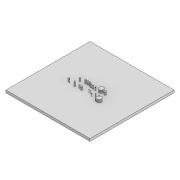
# Autodesk Inventor part: scene7
Saved by Autodesk Inventor 2021 (Build 250183000, 183)
## iProperties
Created: 2022-04-06
Part Number: scene7
Material: Generic
Document SubType Name: Modeling
Designer: Derm
Density: 1 g/cm^3
Appearance: Default
Author: Derm
Autodesk Inventor part; units mm, degrees
ref_plane "YZ Plane" through (0, 0, 0) normal (1, 0, 0) x (0, 1, 0)
ref_plane "XZ Plane" through (0, 0, 0) normal (0, 1, 0) x (-1, 0, 0)
ref_plane "XY Plane" through (0, 0, 0) normal (0, 0, 1) x (1, 0, 0)
sketch "Sketch1" plane through (0, 0, 0) normal (0, 1, 0) x (-1, 0, 0)
  line L0 (-50000, 50000) -> (50000, 50000)
  line L1 (50000, 50000) -> (50000, -50000)
  line L2 (50000, -50000) -> (-50000, -50000)
  line L3 (-50000, -50000) -> (-50000, 50000)
  line L4 (-50000, 50000) -> (50000, -50000) construction
  line L5 (50000, 50000) -> (-50000, -50000) construction
  point P0 (0, 0)
  dimension "d0" = 100000
  dimension "d1" = 100000
  constraints: 12 end point, 2 midpoint, 2 parallel, 1 horizontal, 1 perpendicular
  measures "d0" distance of L1.end L2.end
  measures "d1" distance of L0.end L1.end
extrude "Extrusion1" add sketch "Sketch1" against normal blind 3000
sketch "Sketch2" plane through (0, 0, 0) normal (0, 1, 0) x (1, 0, 0)
  line L0 (50000, 50000) -> (-50000, 50000) projected
  line L1 (-50000, 50000) -> (-50000, -50000) projected
  line L2 (-50000, -50000) -> (50000, -50000) projected
  line L3 (50000, -50000) -> (50000, 50000) projected
  line L4 (50000, 50000) -> (50000, -50000) projected
  line L5 (-50000, -2000) -> (50000, -2000)
  line L6 (50000, -2000) -> (50000, 2000)
  line L7 (50000, 2000) -> (-50000, 2000)
  line L8 (-50000, 2000) -> (-50000, -2000)
  line L9 (-50000, -2000) -> (50000, 2000) construction
  line L10 (50000, -2000) -> (-50000, 2000) construction
  line L11 (5190.5361, 8455.2241) -> (11345.2122, 8455.2241)
  line L12 (11345.2122, 8455.2241) -> (11345.2122, 2832.4339)
  line L13 (11345.2122, 2832.4339) -> (5190.5361, 2832.4339)
  line L14 (5190.5361, 2832.4339) -> (5190.5361, 8455.2241)
  line L15 (5190.5361, 8455.2241) -> (11345.2122, 2832.4339) construction
  line L16 (11345.2122, 8455.2241) -> (5190.5361, 2832.4339) construction
  line L17 (13548.7384, -7995.2366) -> (20995.1366, -7995.2366)
  line L18 (20995.1366, -7995.2366) -> (20995.1366, -2828.3483)
  line L19 (20995.1366, -2828.3483) -> (13548.7384, -2828.3483)
  line L20 (13548.7384, -2828.3483) -> (13548.7384, -7995.2366)
  line L21 (13548.7384, -7995.2366) -> (20995.1366, -2828.3483) construction
  line L22 (20995.1366, -7995.2366) -> (13548.7384, -2828.3483) construction
  line L23 (593.5251, -2562.4055) -> (4772.6262, -2562.4055)
  line L24 (4772.6262, -2562.4055) -> (4772.6262, -3778.1439)
  line L25 (4772.6262, -3778.1439) -> (593.5251, -3778.1439)
  line L26 (593.5251, -3778.1439) -> (593.5251, -2562.4055)
  line L27 (593.5251, -2562.4055) -> (4772.6262, -3778.1439) construction
  line L28 (4772.6262, -2562.4055) -> (593.5251, -3778.1439) construction
  line L29 (-10538.0803, 5605.837) -> (-4079.4695, 5605.837)
  line L30 (-4079.4695, 5605.837) -> (-4079.4695, 3706.2457)
  line L31 (-4079.4695, 3706.2457) -> (-10538.0803, 3706.2457)
  line L32 (-10538.0803, 3706.2457) -> (-10538.0803, 5605.837)
  line L33 (-10538.0803, 5605.837) -> (-4079.4695, 3706.2457) construction
  line L34 (-4079.4695, 5605.837) -> (-10538.0803, 3706.2457) construction
  line L35 (-3357.6248, 4314.115) -> (1581.3128, 4314.115)
  line L36 (1581.3128, 4314.115) -> (1581.3128, 2642.4746)
  line L37 (1581.3128, 2642.4746) -> (-3357.6248, 2642.4746)
  line L38 (-3357.6248, 2642.4746) -> (-3357.6248, 4314.115)
  line L39 (-3357.6248, 4314.115) -> (1581.3128, 2642.4746) construction
  line L40 (1581.3128, 4314.115) -> (-3357.6248, 2642.4746) construction
  line L41 (-9040.7205, -3304.0821) -> (-4779.0471, -3304.0821)
  line L42 (-4779.0471, -3304.0821) -> (-4779.0471, -6275.5798)
  line L43 (-4779.0471, -6275.5798) -> (-9040.7205, -6275.5798)
  line L44 (-9040.7205, -6275.5798) -> (-9040.7205, -3304.0821)
  line L45 (-9040.7205, -3304.0821) -> (-4779.0471, -6275.5798) construction
  line L46 (-4779.0471, -3304.0821) -> (-9040.7205, -6275.5798) construction
  line L47 (12978.8612, 2832.4339) -> (15790.2565, 4086.164)
  line L48 (15790.2565, 4086.164) -> (14919.446, 6038.8907)
  line L49 (14919.446, 6038.8907) -> (12108.0508, 4785.1606)
  line L50 (12108.0508, 4785.1606) -> (12978.8612, 2832.4339)
  line L51 (7237.4094, -5991.9062) -> (11076.909, -4432.894)
  line L52 (11076.909, -4432.894) -> (10571.8855, -3189.1337)
  line L53 (10571.8855, -3189.1337) -> (6732.3859, -4748.1459)
  line L54 (6732.3859, -4748.1459) -> (7237.4094, -5991.9062)
  line L55 (-16072.161, 3808.7972) -> (-15391.3811, 2832.4339)
  line L56 (-15391.3811, 2832.4339) -> (-14124.812, 3715.5628)
  line L57 (-14124.812, 3715.5628) -> (-14805.5919, 4691.9262)
  line L58 (-14805.5919, 4691.9262) -> (-16072.161, 3808.7972)
  line L59 (-23491.5084, -4748.1459) -> (-20999.8327, -7024.4914)
  line L60 (-20999.8327, -7024.4914) -> (-18908.6968, -4735.5451)
  line L61 (-18908.6968, -4735.5451) -> (-21400.3724, -2459.1996)
  line L62 (-21400.3724, -2459.1996) -> (-23491.5084, -4748.1459)
  line L63 (-16105.7388, -3167.2582) -> (-12909.355, -5395.9713)
  line L64 (-12909.355, -5395.9713) -> (-12180.8401, -4351.1472)
  line L65 (-12180.8401, -4351.1472) -> (-15377.224, -2122.4342)
  line L66 (-15377.224, -2122.4342) -> (-16105.7388, -3167.2582)
  line L67 (2445.7903, 4086.164) -> (3479.5334, 2000)
  line L68 (3479.5334, 2000) -> (4246.1072, 2379.8553)
  line L69 (4246.1072, 2379.8553) -> (3212.3641, 4466.0192)
  line L70 (3212.3641, 4466.0192) -> (2445.7903, 4086.164)
  point P0 (0, 0)
  point P1 (8267.8742, 5643.829)
  point P2 (17271.9375, -5411.7924)
  point P3 (2683.0756, -3170.2747)
  point P4 (-7308.7749, 4656.0414)
  point P5 (-888.156, 3478.2948)
  point P6 (-6909.8838, -4789.831)
  dimension "d4" = 4000
  constraints: 132 end point, 27 parallel, 14 midpoint, 13 perpendicular, 7 horizontal, 3 point on line
  measures "d4" distance between parallel lines of L7 L5
extrude "Extrusion2" add sketch "Sketch2" along normal blind 3000 contours L67 L70 L69 L68 | L11 L12 L13 L14 | L20 L19 L18 L17 | L23 L24 L25 L26 | L29 L30 L31 L32 | L35 L36 L37 L38 | L41 L42 L43 L44 | L50 L49 L48 L47 | L54 L53 L52 L51 | L58 L57 L56 L55 | L62 L61 L60 L59 | L66 L65 L64 L63
fillet "Fillet1" [suppressed]
sketch "Sketch3" plane through (0, 0, 0) normal (0, 1, 0) x (1, 0, 0)
  line L0 (-9040.7205, -6275.5798) -> (-9040.7205, -3304.0821) projected
  line L1 (-9040.7205, -3304.0821) -> (-4779.0471, -3304.0821) projected
  line L2 (-4779.0471, -3304.0821) -> (-4779.0471, -6275.5798) projected
  line L3 (-4779.0471, -6275.5798) -> (-9040.7205, -6275.5798) projected
  line L4 (593.5251, -3778.1439) -> (593.5251, -2562.4055) projected
  line L5 (593.5251, -2562.4055) -> (4772.6262, -2562.4055) projected
  line L6 (4772.6262, -2562.4055) -> (4772.6262, -3778.1439) projected
  line L7 (4772.6262, -3778.1439) -> (593.5251, -3778.1439) projected
  line L8 (15790.2565, 4086.164) -> (12978.8612, 2832.4339) projected
  line L9 (12978.8612, 2832.4339) -> (12108.0508, 4785.1606) projected
  line L10 (12108.0508, 4785.1606) -> (14919.446, 6038.8907) projected
  line L11 (14919.446, 6038.8907) -> (15790.2565, 4086.164) projected
  line L12 (5190.5361, 2832.4339) -> (5190.5361, 8455.2241) projected
  line L13 (5190.5361, 8455.2241) -> (11345.2122, 8455.2241) projected
  line L14 (11345.2122, 8455.2241) -> (11345.2122, 2832.4339) projected
  line L15 (11345.2122, 2832.4339) -> (5190.5361, 2832.4339) projected
  line L16 (-3357.6248, 2642.4746) -> (-3357.6248, 4314.115) projected
  line L17 (-3357.6248, 4314.115) -> (1581.3128, 4314.115) projected
  line L18 (1581.3128, 4314.115) -> (1581.3128, 2642.4746) projected
  line L19 (1581.3128, 2642.4746) -> (-3357.6248, 2642.4746) projected
  line L20 (-12909.355, -5395.9713) -> (-16105.7388, -3167.2582) projected
  line L21 (-16105.7388, -3167.2582) -> (-15377.224, -2122.4342) projected
  line L22 (-15377.224, -2122.4342) -> (-12180.8401, -4351.1472) projected
  line L23 (-12180.8401, -4351.1472) -> (-12909.355, -5395.9713) projected
  line L24 (-15391.3811, 2832.4339) -> (-16072.161, 3808.7972) projected
  line L25 (-16072.161, 3808.7972) -> (-14805.5919, 4691.9262) projected
  line L26 (-14805.5919, 4691.9262) -> (-14124.812, 3715.5628) projected
  line L27 (-14124.812, 3715.5628) -> (-15391.3811, 2832.4339) projected
  line L28 (11076.909, -4432.894) -> (7237.4094, -5991.9062) projected
  line L29 (7237.4094, -5991.9062) -> (6732.3859, -4748.1459) projected
  line L30 (6732.3859, -4748.1459) -> (10571.8855, -3189.1337) projected
  line L31 (10571.8855, -3189.1337) -> (11076.909, -4432.894) projected
  line L32 (20995.1366, -7995.2366) -> (13548.7384, -7995.2366) projected
  line L33 (13548.7384, -7995.2366) -> (13548.7384, -2828.3483) projected
  line L34 (13548.7384, -2828.3483) -> (20995.1366, -2828.3483) projected
  line L35 (20995.1366, -2828.3483) -> (20995.1366, -7995.2366) projected
  line L36 (2445.7903, 4086.164) -> (3212.3641, 4466.0192) projected
  line L37 (3212.3641, 4466.0192) -> (4246.1072, 2379.8553) projected
  line L38 (4246.1072, 2379.8553) -> (3479.5334, 2000) projected
  line L39 (3479.5334, 2000) -> (2445.7903, 4086.164) projected
  line L40 (-10538.0803, 3706.2457) -> (-10538.0803, 5605.837) projected
  line L41 (-10538.0803, 5605.837) -> (-4079.4695, 5605.837) projected
  line L42 (-4079.4695, 5605.837) -> (-4079.4695, 3706.2457) projected
  line L43 (-4079.4695, 3706.2457) -> (-10538.0803, 3706.2457) projected
  line L44 (-20999.8327, -7024.4914) -> (-23491.5084, -4748.1459) projected
  line L45 (-23491.5084, -4748.1459) -> (-21400.3724, -2459.1996) projected
  line L46 (-21400.3724, -2459.1996) -> (-18908.6968, -4735.5451) projected
  line L47 (-18908.6968, -4735.5451) -> (-20999.8327, -7024.4914) projected
  line L48 (50000, 50000) -> (-50000, 50000) projected
  line L49 (-50000, 50000) -> (-50000, -50000) projected
  line L50 (-50000, -50000) -> (50000, -50000) projected
  line L51 (50000, -50000) -> (50000, 50000) projected
  circle A0 centre (-21206.9989, -4735.5451) radius 2507.8736
  circle A1 centre (-14179.4153, -3811.0138) radius 1948.3346
  line L52 (-15377.224, -2122.4342) -> (-16105.7388, -3167.2582) projected
  circle A2 centre (-15130.9909, 3808.7972) radius 991.1752
  line L53 (-10538.0803, 3706.2457) -> (-10538.0803, 5605.837) projected
  circle A3 centre (-7308.7749, 7370.1362) radius 4883.9028
  line L54 (1581.3128, 2642.4746) -> (-3357.6248, 2642.4746) projected
  circle A4 centre (-888.156, 6827.5495) radius 4859.3341
  line L55 (4246.1072, 2379.8553) -> (3479.5334, 2000) projected
  circle A5 centre (3345.9488, 3233.0096) radius 1240.2248
  line L56 (5190.5361, 2832.4339) -> (5190.5361, 8455.2241) projected
  circle A6 centre (8267.8742, 8184.0163) radius 6173.2847
  circle A7 centre (14033.4063, 4473.2344) radius 1950.4594
  line L57 (10571.8855, -3189.1337) -> (6732.3859, -4748.1459) projected
  circle A8 centre (8880.1815, -4432.894) radius 2099.7148
  line L58 (4772.6262, -2562.4055) -> (4772.6262, -3778.1439) projected
  circle A9 centre (2683.0756, -3170.2747) radius 2176.1724
  circle A10 centre (-6909.8838, -4789.831) radius 2597.6749
  line L59 (13548.7384, -7995.2366) -> (13548.7384, -2828.3483) projected
  circle A11 centre (16975.0214, -4873.5592) radius 3990.2761
  point P0 (0, 0)
  point P1 (12325.3726, 3531.4739)
  point P2 (14183.1434, 6417.9376)
  point P3 (-16034.8819, -3216.664)
  point P4 (-12980.2119, -5346.5655)
  point P5 (-12287.5612, -4276.7348)
  point P6 (-15270.5029, -2196.8466)
  constraints: 3 centre point, 1 tangent, 27 other
extrude "Extrusion3" [suppressed]
sketch "Sketch4" plane through (0, 0, 0) normal (0, 1, 0) x (1, 0, 0)
  line L0 (50000, 50000) -> (-50000, 50000) projected
  line L1 (-50000, 50000) -> (-50000, -50000) projected
  line L2 (-50000, -50000) -> (50000, -50000) projected
  line L3 (50000, -50000) -> (50000, 50000) projected
  line L4 (11076.909, -4432.894) -> (7237.4094, -5991.9062) projected
  line L5 (7237.4094, -5991.9062) -> (6732.3859, -4748.1459) projected
  line L6 (6732.3859, -4748.1459) -> (10571.8855, -3189.1337) projected
  line L7 (10571.8855, -3189.1337) -> (11076.909, -4432.894) projected
  line L8 (-10538.0803, 3706.2457) -> (-10538.0803, 5605.837) projected
  line L9 (-10538.0803, 5605.837) -> (-4079.4695, 5605.837) projected
  line L10 (-14805.5919, 4691.9262) -> (-14124.812, 3715.5628) projected
  line L11 (-14124.812, 3715.5628) -> (-15391.3811, 2832.4339) projected
  line L12 (-15391.3811, 2832.4339) -> (-16072.161, 3808.7972) projected
  line L13 (593.5251, -3778.1439) -> (593.5251, -2562.4055) projected
  line L14 (4772.6262, -2562.4055) -> (4772.6262, -3778.1439) projected
  line L15 (20995.1366, -7995.2366) -> (13548.7384, -7995.2366) projected
  line L16 (13548.7384, -7995.2366) -> (13548.7384, -2828.3483) projected
  line L17 (13548.7384, -2828.3483) -> (20995.1366, -2828.3483) projected
  line L18 (20995.1366, -2828.3483) -> (20995.1366, -7995.2366) projected
  line L19 (-12909.355, -5395.9713) -> (-16105.7388, -3167.2582) projected
  line L20 (-16105.7388, -3167.2582) -> (-15377.224, -2122.4342) projected
  line L21 (-15377.224, -2122.4342) -> (-12180.8401, -4351.1472) projected
  line L22 (-12180.8401, -4351.1472) -> (-12909.355, -5395.9713) projected
  circle A0 centre (-4095.3087, 1822.3221) radius 119.7331
  circle A1 centre (-3557.0154, -1685.8651) radius 153.3297
  circle A2 centre (1083.4441, 1432.5236) radius 98.3053
  circle A3 centre (5092.8011, 1785.6866) radius 131.4219
  circle A4 centre (5747.1243, -1847.542) radius 169.4608
  circle A5 centre (9343.4621, 1432.5236) radius 127.5966
  circle A6 centre (-7082.9402, 1822.3221) radius 106.718
  circle A7 centre (-7308.7749, -1847.542) radius 87.1079
  circle A8 centre (-10330.2163, 2528.7629) radius 78.0049
  circle A9 centre (-11168.7148, -2334.5281) radius 88.8954
  circle A10 centre (-13446.3785, 2742.5645) radius 100.7642
  line L23 (593.5251, -2562.4055) -> (4772.6262, -2562.4055) projected
  line L24 (4772.6262, -3778.1439) -> (593.5251, -3778.1439) projected
  line L25 (-16072.161, 3808.7972) -> (-14805.5919, 4691.9262) projected
  line L26 (-4079.4695, 5605.837) -> (-4079.4695, 3706.2457) projected
  line L27 (-4079.4695, 3706.2457) -> (-10538.0803, 3706.2457) projected
  point P0 (0, 0)
  constraints: 11 centre point
extrude "Extrusion4" [suppressed]
sketch "Sketch5" plane through (0, 0, 0) normal (0, 1, 0) x (1, 0, 0)
  line L0 (-9040.7205, -6275.5798) -> (-9040.7205, -3304.0821) projected
  line L1 (-9040.7205, -3304.0821) -> (-4779.0471, -3304.0821) projected
  line L2 (-4779.0471, -3304.0821) -> (-4779.0471, -6275.5798) projected
  line L3 (-4779.0471, -6275.5798) -> (-9040.7205, -6275.5798) projected
  line L4 (593.5251, -3778.1439) -> (593.5251, -2562.4055) projected
  line L5 (593.5251, -2562.4055) -> (4772.6262, -2562.4055) projected
  line L6 (4772.6262, -2562.4055) -> (4772.6262, -3778.1439) projected
  line L7 (4772.6262, -3778.1439) -> (593.5251, -3778.1439) projected
  line L8 (15790.2565, 4086.164) -> (12978.8612, 2832.4339) projected
  line L9 (12978.8612, 2832.4339) -> (12108.0508, 4785.1606) projected
  line L10 (12108.0508, 4785.1606) -> (14919.446, 6038.8907) projected
  line L11 (14919.446, 6038.8907) -> (15790.2565, 4086.164) projected
  line L12 (5190.5361, 2832.4339) -> (5190.5361, 8455.2241) projected
  line L13 (5190.5361, 8455.2241) -> (11345.2122, 8455.2241) projected
  line L14 (11345.2122, 8455.2241) -> (11345.2122, 2832.4339) projected
  line L15 (11345.2122, 2832.4339) -> (5190.5361, 2832.4339) projected
  line L16 (-3357.6248, 2642.4746) -> (-3357.6248, 4314.115) projected
  line L17 (-3357.6248, 4314.115) -> (1581.3128, 4314.115) projected
  line L18 (1581.3128, 4314.115) -> (1581.3128, 2642.4746) projected
  line L19 (1581.3128, 2642.4746) -> (-3357.6248, 2642.4746) projected
  line L20 (-12909.355, -5395.9713) -> (-16105.7388, -3167.2582) projected
  line L21 (-16105.7388, -3167.2582) -> (-15377.224, -2122.4342) projected
  line L22 (-15377.224, -2122.4342) -> (-12180.8401, -4351.1472) projected
  line L23 (-12180.8401, -4351.1472) -> (-12909.355, -5395.9713) projected
  line L24 (-15391.3811, 2832.4339) -> (-16072.161, 3808.7972) projected
  line L25 (-16072.161, 3808.7972) -> (-14805.5919, 4691.9262) projected
  line L26 (-14805.5919, 4691.9262) -> (-14124.812, 3715.5628) projected
  line L27 (-14124.812, 3715.5628) -> (-15391.3811, 2832.4339) projected
  line L28 (11076.909, -4432.894) -> (7237.4094, -5991.9062) projected
  line L29 (7237.4094, -5991.9062) -> (6732.3859, -4748.1459) projected
  line L30 (6732.3859, -4748.1459) -> (10571.8855, -3189.1337) projected
  line L31 (10571.8855, -3189.1337) -> (11076.909, -4432.894) projected
  line L32 (20995.1366, -7995.2366) -> (13548.7384, -7995.2366) projected
  line L33 (13548.7384, -7995.2366) -> (13548.7384, -2828.3483) projected
  line L34 (13548.7384, -2828.3483) -> (20995.1366, -2828.3483) projected
  line L35 (20995.1366, -2828.3483) -> (20995.1366, -7995.2366) projected
  line L36 (2445.7903, 4086.164) -> (3212.3641, 4466.0192) projected
  line L37 (3212.3641, 4466.0192) -> (4246.1072, 2379.8553) projected
  line L38 (4246.1072, 2379.8553) -> (3479.5334, 2000) projected
  line L39 (3479.5334, 2000) -> (2445.7903, 4086.164) projected
  line L40 (-10538.0803, 3706.2457) -> (-10538.0803, 5605.837) projected
  line L41 (-10538.0803, 5605.837) -> (-4079.4695, 5605.837) projected
  line L42 (-4079.4695, 5605.837) -> (-4079.4695, 3706.2457) projected
  line L43 (-4079.4695, 3706.2457) -> (-10538.0803, 3706.2457) projected
  line L44 (-20999.8327, -7024.4914) -> (-23491.5084, -4748.1459) projected
  line L45 (-23491.5084, -4748.1459) -> (-21400.3724, -2459.1996) projected
  line L46 (-21400.3724, -2459.1996) -> (-18908.6968, -4735.5451) projected
  line L47 (-18908.6968, -4735.5451) -> (-20999.8327, -7024.4914) projected
  line L48 (50000, 50000) -> (-50000, 50000) projected
  line L49 (-50000, 50000) -> (-50000, -50000) projected
  line L50 (-50000, -50000) -> (50000, -50000) projected
  line L51 (50000, -50000) -> (50000, 50000) projected
  point P0 (0, 0)
sketch "Sketch6" plane through (0, 0, 0) normal (0, 1, 0) x (1, 0, 0)
  line L0 (-50000, 50000) -> (50000, 50000) projected
  line L1 (50000, 50000) -> (50000, -50000) projected
  line L2 (50000, -50000) -> (-50000, -50000) projected
  line L3 (-50000, -50000) -> (-50000, 50000) projected
  point P0 (0, 0)
extrude "Extrusion5" cut sketch "Sketch6" along normal through all
sketch "Sketch7" plane through (0, 0, 0) normal (0, 1, 0) x (1, 0, 0)
  circle A0 centre (-9978.6465, 4710.7622) radius 1023.7749
  circle A1 centre (-7214.3022, 4710.7622) radius 1027.6511
  circle A2 centre (-4676.9421, 4645.9096) radius 971.4959
  circle A3 centre (-2301.7138, 3486.6684) radius 789.6327
  circle A4 centre (178.9002, 3486.6684) radius 790.2982
  circle A5 centre (3137.8025, 3770.3988) radius 397.5532
  circle A6 centre (3729.5829, 2586.8378) radius 460.4367
  circle A7 centre (8196.3586, 5393.018) radius 2710.5154
  circle A8 centre (13563.4865, 4461.9856) radius 1159.7903
  circle A9 centre (4190.0196, -3150.5735) radius 440.1512
  circle A10 centre (1870.8149, -3013.657) radius 332.7122
  circle A11 centre (-5385.7611, -4410.2056) radius 1098.5138
  circle A12 centre (-8616.9912, -4026.8393) radius 723.487
  circle A13 centre (-15325.9011, -3013.657) radius 545.6085
  circle A14 centre (-13354.3031, -4750.3263) radius 996.0356
  circle A15 centre (-15325.9011, 3302.1952) radius 908.0305
  circle A16 centre (-21706.2113, -3559.2655) radius 912.2416
  circle A17 centre (-19953.6798, -4471.5071) radius 383.3663
  circle A18 centre (7457.0094, -5231.7048) radius 377.825
  circle A19 centre (10332.2565, -3559.2655) radius 587.9445
  circle A20 centre (13946.8529, -3303.3523) radius 501.3338
  circle A21 centre (14448.1867, -7230.6861) radius 816.7974
  circle A22 centre (16603.0335, -5609.5298) radius 2771.4161
  point P0 (0, 0)
  point P1 (14976.6122, -7853.522)
  point P2 (13996.1945, -6550.3472)
  constraints: 23 centre point
extrude "Extrusion6" add sketch "Sketch7" along normal blind 3000
body "Solid1"
